Autodesk Inventor part; units mm, degrees
(part 2 of 2)
sketch "Sketch21" plane through (-13, -6, 11) normal (0, 0, 1) x (1, 0, 0)
  line L0 (3, 1.5332) -> (-3, 1.5332)
  arc A0 (3, 1.5332) -> (-3, 1.5332) centre (0, 0) ccw
  circle A1 centre (0, 0) radius 3.5 projected
  line L1 (2.0687, 0.6882) -> (2.0687, -0.0132) construction
  line L2 (2.0687, -0.0132) -> (1.4411, -0.0132) construction
  line L3 (1.4411, -0.0132) -> (1.4411, 0.6882) construction
  line L4 (1.4411, 0.6882) -> (2.0687, 0.6882) construction
  line L5 (11, 13.9476) -> (5, 13.9476)
  arc A2 (11, 13.9476) -> (5, 13.9476) centre (8, 12.4145) ccw
  line L6 (10.0687, 12.6882) -> (10.0687, 11.9868) construction
  line L7 (10.0687, 11.9868) -> (9.4411, 11.9868) construction
  line L8 (9.4411, 11.9868) -> (9.4411, 12.6882) construction
  line L9 (9.4411, 12.6882) -> (10.0687, 12.6882) construction
  line L10 (3, 1.5332) -> (-3, 1.5332)
  arc A3 (3, 1.5332) -> (-3, 1.5332) centre (0, 0) ccw
  line L11 (11, 13.9476) -> (5, 13.9476)
  arc A4 (11, 13.9476) -> (5, 13.9476) centre (8, 12.4145) ccw
  line L12 (1.0216, -0.0191) -> (1.0216, 0.6134)
  line L13 (1.0216, 0.6134) -> (1.1671, 0.6134)
  spline S0 degree 2 poles (1.1671, 0.6134) (1.2311, 0.5452) (1.3499, 0.4239) (1.4139, 0.3657) knots 0 0 0 1 2 2 2
  spline S1 degree 2 poles (1.4139, 0.3657) (1.5427, 0.2485) (1.6973, 0.1629) (1.7795, 0.1629) knots 0 0 0 1 2 2 2
  spline S2 degree 2 poles (1.7795, 0.1629) (1.8228, 0.1629) (1.8876, 0.1895) (1.9084, 0.2136) knots 0 0 0 1 2 2 2
  spline S3 degree 2 poles (1.9084, 0.2136) (1.9291, 0.2377) (1.9499, 0.3009) (1.9499, 0.3391) knots 0 0 0 1 2 2 2
  spline S4 degree 2 poles (1.9499, 0.3391) (1.9499, 0.3757) (1.9316, 0.4505) (1.9175, 0.4845) knots 0 0 0 1 2 2 2
  spline S5 degree 2 poles (1.9175, 0.4845) (1.9059, 0.5136) (1.8726, 0.5677) (1.861, 0.5843) knots 0 0 0 1 2 2 2
  line L14 (1.861, 0.5843) -> (1.861, 0.5918)
  line L15 (1.861, 0.5918) -> (2.0073, 0.5918)
  spline S6 degree 2 poles (2.0073, 0.5918) (2.028, 0.5494) (2.0687, 0.3973) (2.0687, 0.3291) knots 0 0 0 1 2 2 2
  spline S7 degree 2 poles (2.0687, 0.3291) (2.0687, 0.1854) (1.9167, 0.0233) (1.787, 0.0233) knots 0 0 0 1 2 2 2
  spline S8 degree 2 poles (1.787, 0.0233) (1.7264, 0.0233) (1.625, 0.0516) (1.5818, 0.0765) knots 0 0 0 1 2 2 2
  spline S9 degree 2 poles (1.5818, 0.0765) (1.5369, 0.1014) (1.4488, 0.1737) (1.4064, 0.2136) knots 0 0 0 1 2 2 2
  spline S10 degree 2 poles (1.4064, 0.2136) (1.3358, 0.2784) (1.1845, 0.4372) (1.1405, 0.4845) knots 0 0 0 1 2 2 2
  line L16 (1.1405, 0.4845) -> (1.1405, -0.0191)
  line L17 (1.1405, -0.0191) -> (1.0216, -0.0191)
  line L18 (1.0216, -0.7886) -> (1.0216, -0.1562)
  line L19 (1.0216, -0.1562) -> (1.1671, -0.1562)
  spline S11 degree 2 poles (1.1671, -0.1562) (1.2311, -0.2243) (1.3499, -0.3457) (1.4139, -0.4038) knots 0 0 0 1 2 2 2
  spline S12 degree 2 poles (1.4139, -0.4038) (1.5427, -0.521) (1.6973, -0.6066) (1.7795, -0.6066) knots 0 0 0 1 2 2 2
  spline S13 degree 2 poles (1.7795, -0.6066) (1.8228, -0.6066) (1.8876, -0.58) (1.9084, -0.5559) knots 0 0 0 1 2 2 2
  spline S14 degree 2 poles (1.9084, -0.5559) (1.9291, -0.5318) (1.9499, -0.4687) (1.9499, -0.4304) knots 0 0 0 1 2 2 2
  spline S15 degree 2 poles (1.9499, -0.4304) (1.9499, -0.3939) (1.9316, -0.3191) (1.9175, -0.285) knots 0 0 0 1 2 2 2
  spline S16 degree 2 poles (1.9175, -0.285) (1.9059, -0.2559) (1.8726, -0.2019) (1.861, -0.1853) knots 0 0 0 1 2 2 2
  line L20 (1.861, -0.1853) -> (1.861, -0.1778)
  line L21 (1.861, -0.1778) -> (2.0073, -0.1778)
  spline S17 degree 2 poles (2.0073, -0.1778) (2.028, -0.2202) (2.0687, -0.3723) (2.0687, -0.4404) knots 0 0 0 1 2 2 2
  spline S18 degree 2 poles (2.0687, -0.4404) (2.0687, -0.5842) (1.9167, -0.7462) (1.787, -0.7462) knots 0 0 0 1 2 2 2
  spline S19 degree 2 poles (1.787, -0.7462) (1.7264, -0.7462) (1.625, -0.718) (1.5818, -0.693) knots 0 0 0 1 2 2 2
  spline S20 degree 2 poles (1.5818, -0.693) (1.5369, -0.6681) (1.4488, -0.5958) (1.4064, -0.5559) knots 0 0 0 1 2 2 2
  spline S21 degree 2 poles (1.4064, -0.5559) (1.3358, -0.4911) (1.1845, -0.3324) (1.1405, -0.285) knots 0 0 0 1 2 2 2
  line L22 (1.1405, -0.285) -> (1.1405, -0.7886)
  line L23 (1.1405, -0.7886) -> (1.0216, -0.7886)
  spline S22 degree 2 poles (1.5344, -1.564) (1.2585, -1.564) (1, -1.4036) (1, -1.2365) knots 0 0 0 1 2 2 2
  spline S23 degree 2 poles (1, -1.2365) (1, -1.067) (1.2635, -0.9083) (1.5336, -0.9083) knots 0 0 0 1 2 2 2
  spline S24 degree 2 poles (1.5336, -0.9083) (1.8111, -0.9083) (2.0679, -1.0687) (2.0679, -1.2365) knots 0 0 0 1 2 2 2
  spline S25 degree 2 poles (2.0679, -1.2365) (2.0679, -1.4052) (1.802, -1.564) (1.5344, -1.564) knots 0 0 0 1 2 2 2
  spline S26 degree 2 poles (1.2219, -1.3878) (1.2726, -1.4077) (1.4288, -1.4243) (1.5344, -1.4243) knots 0 0 0 1 2 2 2
  spline S27 degree 2 poles (1.5344, -1.4243) (1.6399, -1.4243) (1.7953, -1.4077) (1.8477, -1.3869) knots 0 0 0 1 2 2 2
  spline S28 degree 2 poles (1.8477, -1.3869) (1.9, -1.3662) (1.9541, -1.2939) (1.9541, -1.2365) knots 0 0 0 1 2 2 2
  spline S29 degree 2 poles (1.9541, -1.2365) (1.9541, -1.1792) (1.9, -1.1052) (1.846, -1.0836) knots 0 0 0 1 2 2 2
  spline S30 degree 2 poles (1.846, -1.0836) (1.7937, -1.0628) (1.6341, -1.0479) (1.5336, -1.0479) knots 0 0 0 1 2 2 2
  spline S31 degree 2 poles (1.5336, -1.0479) (1.4255, -1.0479) (1.2809, -1.0612) (1.2244, -1.0828) knots 0 0 0 1 2 2 2
  spline S32 degree 2 poles (1.2244, -1.0828) (1.1712, -1.1027) (1.1139, -1.1767) (1.1139, -1.2365) knots 0 0 0 1 2 2 2
  spline S33 degree 2 poles (1.1139, -1.2365) (1.1139, -1.293) (1.1679, -1.367) (1.2219, -1.3878) knots 0 0 0 1 2 2 2
  spline S34 degree 2 poles (0.2615, 0.3366) (0.2615, 0.374) (0.2432, 0.448) (0.229, 0.4837) knots 0 0 0 1 2 2 2
  spline S35 degree 2 poles (0.229, 0.4837) (0.2149, 0.517) (0.185, 0.566) (0.1717, 0.5851) knots 0 0 0 1 2 2 2
  line L24 (0.1717, 0.5851) -> (0.1717, 0.5934)
  line L25 (0.1717, 0.5934) -> (0.3171, 0.5934)
  spline S36 degree 2 poles (0.3171, 0.5934) (0.3412, 0.5485) (0.3803, 0.3948) (0.3803, 0.3258) knots 0 0 0 1 2 2 2
  spline S37 degree 2 poles (0.3803, 0.3258) (0.3803, 0.256) (0.352, 0.1521) (0.3221, 0.1097) knots 0 0 0 1 2 2 2
  spline S38 degree 2 poles (0.3221, 0.1097) (0.2897, 0.0649) (0.1958, 0.0183) (0.1326, 0.0183) knots 0 0 0 1 2 2 2
  spline S39 degree 2 poles (0.1326, 0.0183) (0.0479, 0.0183) (-0.0801, 0.1297) (-0.0967, 0.2078) knots 0 0 0 1 2 2 2
  line L26 (-0.0967, 0.2078) -> (-0.1067, 0.2078)
  spline S40 degree 2 poles (-0.1067, 0.2078) (-0.1133, 0.1754) (-0.1433, 0.1014) (-0.1732, 0.0699) knots 0 0 0 1 2 2 2
  spline S41 degree 2 poles (-0.1732, 0.0699) (-0.2023, 0.0383) (-0.2953, -0.0016) (-0.3627, -0.0016) knots 0 0 0 1 2 2 2
  spline S42 degree 2 poles (-0.3627, -0.0016) (-0.4316, -0.0016) (-0.5488, 0.0458) (-0.5937, 0.089) knots 0 0 0 1 2 2 2
  spline S43 degree 2 poles (-0.5937, 0.089) (-0.6402, 0.1338) (-0.6884, 0.261) (-0.6884, 0.3416) knots 0 0 0 1 2 2 2
  spline S44 degree 2 poles (-0.6884, 0.3416) (-0.6884, 0.4189) (-0.651, 0.5701) (-0.6253, 0.6217) knots 0 0 0 1 2 2 2
  line L27 (-0.6253, 0.6217) -> (-0.4798, 0.6217)
  line L28 (-0.4798, 0.6217) -> (-0.4798, 0.6117)
  spline S45 degree 2 poles (-0.4798, 0.6117) (-0.5114, 0.5685) (-0.5696, 0.4222) (-0.5696, 0.3499) knots 0 0 0 1 2 2 2
  spline S46 degree 2 poles (-0.5696, 0.3499) (-0.5696, 0.3075) (-0.543, 0.2228) (-0.5122, 0.1945) knots 0 0 0 1 2 2 2
  spline S47 degree 2 poles (-0.5122, 0.1945) (-0.4815, 0.1671) (-0.4084, 0.138) (-0.3527, 0.138) knots 0 0 0 1 2 2 2
  spline S48 degree 2 poles (-0.3527, 0.138) (-0.297, 0.138) (-0.2247, 0.1704) (-0.2039, 0.1995) knots 0 0 0 1 2 2 2
  spline S49 degree 2 poles (-0.2039, 0.1995) (-0.1832, 0.2286) (-0.1674, 0.3075) (-0.1674, 0.3541) knots 0 0 0 1 2 2 2
  line L29 (-0.1674, 0.3541) -> (-0.1674, 0.4122)
  line L30 (-0.1674, 0.4122) -> (-0.0535, 0.4122)
  line L31 (-0.0535, 0.4122) -> (-0.0535, 0.3665)
  spline S50 degree 2 poles (-0.0535, 0.3665) (-0.0535, 0.2743) (0.0346, 0.1579) (0.1185, 0.1579) knots 0 0 0 1 2 2 2
  spline S51 degree 2 poles (0.1185, 0.1579) (0.1576, 0.1579) (0.2133, 0.1879) (0.2299, 0.212) knots 0 0 0 1 2 2 2
  spline S52 degree 2 poles (0.2299, 0.212) (0.2473, 0.2377) (0.2615, 0.3009) (0.2615, 0.3366) knots 0 0 0 1 2 2 2
  spline S53 degree 2 poles (-0.3411, -0.7778) (-0.415, -0.7778) (-0.5413, -0.7304) (-0.5879, -0.6872) knots 0 0 0 1 2 2 2
  spline S54 degree 2 poles (-0.5879, -0.6872) (-0.6344, -0.644) (-0.6884, -0.5152) (-0.6884, -0.4354) knots 0 0 0 1 2 2 2
  spline S55 degree 2 poles (-0.6884, -0.4354) (-0.6884, -0.3623) (-0.656, -0.2193) (-0.6303, -0.167) knots 0 0 0 1 2 2 2
  line L32 (-0.6303, -0.167) -> (-0.4848, -0.167)
  line L33 (-0.4848, -0.167) -> (-0.4848, -0.177)
  spline S56 degree 2 poles (-0.4848, -0.177) (-0.4965, -0.1927) (-0.5264, -0.2518) (-0.5397, -0.2875) knots 0 0 0 1 2 2 2
  spline S57 degree 2 poles (-0.5397, -0.2875) (-0.5538, -0.3282) (-0.5696, -0.3955) (-0.5696, -0.4379) knots 0 0 0 1 2 2 2
  spline S58 degree 2 poles (-0.5696, -0.4379) (-0.5696, -0.4795) (-0.5397, -0.5576) (-0.5073, -0.5858) knots 0 0 0 1 2 2 2
  spline S59 degree 2 poles (-0.5073, -0.5858) (-0.4765, -0.6116) (-0.3951, -0.6382) (-0.3402, -0.6382) knots 0 0 0 1 2 2 2
  spline S60 degree 2 poles (-0.3402, -0.6382) (-0.2854, -0.6382) (-0.2156, -0.6083) (-0.1923, -0.58) knots 0 0 0 1 2 2 2
  spline S61 degree 2 poles (-0.1923, -0.58) (-0.1665, -0.5509) (-0.1449, -0.4645) (-0.1449, -0.4121) knots 0 0 0 1 2 2 2
  spline S62 degree 2 poles (-0.1449, -0.4121) (-0.1449, -0.3556) (-0.1624, -0.2434) (-0.1699, -0.2094) knots 0 0 0 1 2 2 2
  line L34 (-0.1699, -0.2094) -> (0.3587, -0.2094)
  line L35 (0.3587, -0.2094) -> (0.3587, -0.772)
  line L36 (0.3587, -0.772) -> (0.2382, -0.772)
  line L37 (0.2382, -0.772) -> (0.2382, -0.3415)
  line L38 (0.2382, -0.3415) -> (-0.0352, -0.3415)
  spline S63 degree 2 poles (-0.0352, -0.3415) (-0.0319, -0.3664) (-0.0294, -0.4146) (-0.0294, -0.4346) knots 0 0 0 1 2 2 2
  spline S64 degree 2 poles (-0.0294, -0.4346) (-0.0294, -0.5135) (-0.0552, -0.6224) (-0.0934, -0.6723) knots 0 0 0 1 2 2 2
  spline S65 degree 2 poles (-0.0934, -0.6723) (-0.1316, -0.723) (-0.248, -0.7778) (-0.3411, -0.7778) knots 0 0 0 1 2 2 2
  line L39 (0.3587, -1.6986) -> (-0.6668, -1.3454)
  line L40 (-0.6668, -1.3454) -> (-0.6668, -1.1983)
  line L41 (-0.6668, -1.1983) -> (0.3587, -0.8451)
  line L42 (0.3587, -0.8451) -> (0.3587, -0.9914)
  line L43 (0.3587, -0.9914) -> (-0.4931, -1.2756)
  line L44 (-0.4931, -1.2756) -> (0.3587, -1.5598)
  line L45 (0.3587, -1.5598) -> (0.3587, -1.6986)
  spline S66 degree 2 poles (-2.3769, 0.2261) (-2.3769, 0.3167) (-2.3295, 0.4513) (-2.2821, 0.4987) knots 0 0 0 1 2 2 2
  spline S67 degree 2 poles (-2.2821, 0.4987) (-2.229, 0.5527) (-2.0794, 0.5967) (-1.9697, 0.5967) knots 0 0 0 1 2 2 2
  line L46 (-1.9697, 0.5967) -> (-1.3298, 0.5967)
  line L47 (-1.3298, 0.5967) -> (-1.3298, 0.4604)
  line L48 (-1.3298, 0.4604) -> (-1.9697, 0.4604)
  spline S68 degree 2 poles (-1.9697, 0.4604) (-2.0411, 0.4604) (-2.1375, 0.4422) (-2.1766, 0.4164) knots 0 0 0 1 2 2 2
  spline S69 degree 2 poles (-2.1766, 0.4164) (-2.2182, 0.389) (-2.2605, 0.2942) (-2.2605, 0.2261) knots 0 0 0 1 2 2 2
  spline S70 degree 2 poles (-2.2605, 0.2261) (-2.2605, 0.1621) (-2.2182, 0.0624) (-2.1766, 0.035) knots 0 0 0 1 2 2 2
  spline S71 degree 2 poles (-2.1766, 0.035) (-2.1375, 0.0092) (-2.042, -0.0091) (-1.973, -0.0091) knots 0 0 0 1 2 2 2
  line L49 (-1.973, -0.0091) -> (-1.3298, -0.0091)
  line L50 (-1.3298, -0.0091) -> (-1.3298, -0.1454)
  line L51 (-1.3298, -0.1454) -> (-1.9697, -0.1454)
  spline S72 degree 2 poles (-1.9697, -0.1454) (-2.0769, -0.1454) (-2.2298, -0.1022) (-2.2821, -0.0473) knots 0 0 0 1 2 2 2
  spline S73 degree 2 poles (-2.2821, -0.0473) (-2.3303, 0.0017) (-2.3769, 0.1314) (-2.3769, 0.2261) knots 0 0 0 1 2 2 2
  line L52 (-2.3553, -0.58) -> (-1.4511, -0.58)
  line L53 (-1.4511, -0.58) -> (-1.4511, -0.236)
  line L54 (-1.4511, -0.236) -> (-1.3298, -0.236)
  line L55 (-1.3298, -0.236) -> (-1.3298, -1.0604)
  line L56 (-1.3298, -1.0604) -> (-1.4511, -1.0604)
  line L57 (-1.4511, -1.0604) -> (-1.4511, -0.7163)
  line L58 (-1.4511, -0.7163) -> (-2.3553, -0.7163)
  line L59 (-2.3553, -0.7163) -> (-2.3553, -0.58)
  line L60 (9.0216, 11.9809) -> (9.0216, 12.6134)
  line L61 (9.0216, 12.6134) -> (9.1671, 12.6134)
  spline S74 degree 2 poles (9.1671, 12.6134) (9.2311, 12.5452) (9.3499, 12.4239) (9.4139, 12.3657) knots 0 0 0 1 2 2 2
  spline S75 degree 2 poles (9.4139, 12.3657) (9.5427, 12.2485) (9.6973, 12.1629) (9.7795, 12.1629) knots 0 0 0 1 2 2 2
  spline S76 degree 2 poles (9.7795, 12.1629) (9.8228, 12.1629) (9.8876, 12.1895) (9.9084, 12.2136) knots 0 0 0 1 2 2 2
  spline S77 degree 2 poles (9.9084, 12.2136) (9.9291, 12.2377) (9.9499, 12.3009) (9.9499, 12.3391) knots 0 0 0 1 2 2 2
  spline S78 degree 2 poles (9.9499, 12.3391) (9.9499, 12.3757) (9.9316, 12.4505) (9.9175, 12.4845) knots 0 0 0 1 2 2 2
  spline S79 degree 2 poles (9.9175, 12.4845) (9.9059, 12.5136) (9.8726, 12.5677) (9.861, 12.5843) knots 0 0 0 1 2 2 2
  line L62 (9.861, 12.5843) -> (9.861, 12.5918)
  line L63 (9.861, 12.5918) -> (10.0073, 12.5918)
  spline S80 degree 2 poles (10.0073, 12.5918) (10.028, 12.5494) (10.0687, 12.3973) (10.0687, 12.3291) knots 0 0 0 1 2 2 2
  spline S81 degree 2 poles (10.0687, 12.3291) (10.0687, 12.1854) (9.9167, 12.0233) (9.787, 12.0233) knots 0 0 0 1 2 2 2
  spline S82 degree 2 poles (9.787, 12.0233) (9.7264, 12.0233) (9.625, 12.0516) (9.5818, 12.0765) knots 0 0 0 1 2 2 2
  spline S83 degree 2 poles (9.5818, 12.0765) (9.5369, 12.1014) (9.4488, 12.1737) (9.4064, 12.2136) knots 0 0 0 1 2 2 2
  spline S84 degree 2 poles (9.4064, 12.2136) (9.3358, 12.2784) (9.1845, 12.4372) (9.1405, 12.4845) knots 0 0 0 1 2 2 2
  line L64 (9.1405, 12.4845) -> (9.1405, 11.9809)
  line L65 (9.1405, 11.9809) -> (9.0216, 11.9809)
  line L66 (9.0216, 11.2114) -> (9.0216, 11.8438)
  line L67 (9.0216, 11.8438) -> (9.1671, 11.8438)
  spline S85 degree 2 poles (9.1671, 11.8438) (9.2311, 11.7757) (9.3499, 11.6543) (9.4139, 11.5962) knots 0 0 0 1 2 2 2
  spline S86 degree 2 poles (9.4139, 11.5962) (9.5427, 11.479) (9.6973, 11.3934) (9.7795, 11.3934) knots 0 0 0 1 2 2 2
  spline S87 degree 2 poles (9.7795, 11.3934) (9.8228, 11.3934) (9.8876, 11.42) (9.9084, 11.4441) knots 0 0 0 1 2 2 2
  spline S88 degree 2 poles (9.9084, 11.4441) (9.9291, 11.4682) (9.9499, 11.5313) (9.9499, 11.5696) knots 0 0 0 1 2 2 2
  spline S89 degree 2 poles (9.9499, 11.5696) (9.9499, 11.6061) (9.9316, 11.6809) (9.9175, 11.715) knots 0 0 0 1 2 2 2
  spline S90 degree 2 poles (9.9175, 11.715) (9.9059, 11.7441) (9.8726, 11.7981) (9.861, 11.8147) knots 0 0 0 1 2 2 2
  line L68 (9.861, 11.8147) -> (9.861, 11.8222)
  line L69 (9.861, 11.8222) -> (10.0073, 11.8222)
  spline S91 degree 2 poles (10.0073, 11.8222) (10.028, 11.7798) (10.0687, 11.6277) (10.0687, 11.5596) knots 0 0 0 1 2 2 2
  spline S92 degree 2 poles (10.0687, 11.5596) (10.0687, 11.4158) (9.9167, 11.2538) (9.787, 11.2538) knots 0 0 0 1 2 2 2
  spline S93 degree 2 poles (9.787, 11.2538) (9.7264, 11.2538) (9.625, 11.282) (9.5818, 11.307) knots 0 0 0 1 2 2 2
  spline S94 degree 2 poles (9.5818, 11.307) (9.5369, 11.3319) (9.4488, 11.4042) (9.4064, 11.4441) knots 0 0 0 1 2 2 2
  spline S95 degree 2 poles (9.4064, 11.4441) (9.3358, 11.5089) (9.1845, 11.6676) (9.1405, 11.715) knots 0 0 0 1 2 2 2
  line L70 (9.1405, 11.715) -> (9.1405, 11.2114)
  line L71 (9.1405, 11.2114) -> (9.0216, 11.2114)
  spline S96 degree 2 poles (9.5344, 10.436) (9.2585, 10.436) (9, 10.5964) (9, 10.7635) knots 0 0 0 1 2 2 2
  spline S97 degree 2 poles (9, 10.7635) (9, 10.933) (9.2635, 11.0917) (9.5336, 11.0917) knots 0 0 0 1 2 2 2
  spline S98 degree 2 poles (9.5336, 11.0917) (9.8111, 11.0917) (10.0679, 10.9313) (10.0679, 10.7635) knots 0 0 0 1 2 2 2
  spline S99 degree 2 poles (10.0679, 10.7635) (10.0679, 10.5948) (9.802, 10.436) (9.5344, 10.436) knots 0 0 0 1 2 2 2
  spline S100 degree 2 poles (9.2219, 10.6122) (9.2726, 10.5923) (9.4288, 10.5757) (9.5344, 10.5757) knots 0 0 0 1 2 2 2
  spline S101 degree 2 poles (9.5344, 10.5757) (9.6399, 10.5757) (9.7953, 10.5923) (9.8477, 10.6131) knots 0 0 0 1 2 2 2
  spline S102 degree 2 poles (9.8477, 10.6131) (9.9, 10.6338) (9.9541, 10.7061) (9.9541, 10.7635) knots 0 0 0 1 2 2 2
  spline S103 degree 2 poles (9.9541, 10.7635) (9.9541, 10.8208) (9.9, 10.8948) (9.846, 10.9164) knots 0 0 0 1 2 2 2
  spline S104 degree 2 poles (9.846, 10.9164) (9.7937, 10.9372) (9.6341, 10.9521) (9.5336, 10.9521) knots 0 0 0 1 2 2 2
  spline S105 degree 2 poles (9.5336, 10.9521) (9.4255, 10.9521) (9.2809, 10.9388) (9.2244, 10.9172) knots 0 0 0 1 2 2 2
  spline S106 degree 2 poles (9.2244, 10.9172) (9.1712, 10.8973) (9.1139, 10.8233) (9.1139, 10.7635) knots 0 0 0 1 2 2 2
  spline S107 degree 2 poles (9.1139, 10.7635) (9.1139, 10.707) (9.1679, 10.633) (9.2219, 10.6122) knots 0 0 0 1 2 2 2
  spline S108 degree 2 poles (8.2615, 12.3366) (8.2615, 12.374) (8.2432, 12.448) (8.229, 12.4837) knots 0 0 0 1 2 2 2
  spline S109 degree 2 poles (8.229, 12.4837) (8.2149, 12.517) (8.185, 12.566) (8.1717, 12.5851) knots 0 0 0 1 2 2 2
  line L72 (8.1717, 12.5851) -> (8.1717, 12.5934)
  line L73 (8.1717, 12.5934) -> (8.3171, 12.5934)
  spline S110 degree 2 poles (8.3171, 12.5934) (8.3412, 12.5485) (8.3803, 12.3948) (8.3803, 12.3258) knots 0 0 0 1 2 2 2
  spline S111 degree 2 poles (8.3803, 12.3258) (8.3803, 12.256) (8.352, 12.1521) (8.3221, 12.1097) knots 0 0 0 1 2 2 2
  spline S112 degree 2 poles (8.3221, 12.1097) (8.2897, 12.0649) (8.1958, 12.0183) (8.1326, 12.0183) knots 0 0 0 1 2 2 2
  spline S113 degree 2 poles (8.1326, 12.0183) (8.0479, 12.0183) (7.9199, 12.1297) (7.9033, 12.2078) knots 0 0 0 1 2 2 2
  line L74 (7.9033, 12.2078) -> (7.8933, 12.2078)
  spline S114 degree 2 poles (7.8933, 12.2078) (7.8867, 12.1754) (7.8567, 12.1014) (7.8268, 12.0699) knots 0 0 0 1 2 2 2
  spline S115 degree 2 poles (7.8268, 12.0699) (7.7977, 12.0383) (7.7047, 11.9984) (7.6373, 11.9984) knots 0 0 0 1 2 2 2
  spline S116 degree 2 poles (7.6373, 11.9984) (7.5684, 11.9984) (7.4512, 12.0458) (7.4063, 12.089) knots 0 0 0 1 2 2 2
  spline S117 degree 2 poles (7.4063, 12.089) (7.3598, 12.1338) (7.3116, 12.261) (7.3116, 12.3416) knots 0 0 0 1 2 2 2
  spline S118 degree 2 poles (7.3116, 12.3416) (7.3116, 12.4189) (7.349, 12.5701) (7.3747, 12.6217) knots 0 0 0 1 2 2 2
  line L75 (7.3747, 12.6217) -> (7.5202, 12.6217)
  line L76 (7.5202, 12.6217) -> (7.5202, 12.6117)
  spline S119 degree 2 poles (7.5202, 12.6117) (7.4886, 12.5685) (7.4304, 12.4222) (7.4304, 12.3499) knots 0 0 0 1 2 2 2
  spline S120 degree 2 poles (7.4304, 12.3499) (7.4304, 12.3075) (7.457, 12.2228) (7.4878, 12.1945) knots 0 0 0 1 2 2 2
  spline S121 degree 2 poles (7.4878, 12.1945) (7.5185, 12.1671) (7.5916, 12.138) (7.6473, 12.138) knots 0 0 0 1 2 2 2
  spline S122 degree 2 poles (7.6473, 12.138) (7.703, 12.138) (7.7753, 12.1704) (7.7961, 12.1995) knots 0 0 0 1 2 2 2
  spline S123 degree 2 poles (7.7961, 12.1995) (7.8168, 12.2286) (7.8326, 12.3075) (7.8326, 12.3541) knots 0 0 0 1 2 2 2
  line L77 (7.8326, 12.3541) -> (7.8326, 12.4122)
  line L78 (7.8326, 12.4122) -> (7.9465, 12.4122)
  line L79 (7.9465, 12.4122) -> (7.9465, 12.3665)
  spline S124 degree 2 poles (7.9465, 12.3665) (7.9465, 12.2743) (8.0346, 12.1579) (8.1185, 12.1579) knots 0 0 0 1 2 2 2
  spline S125 degree 2 poles (8.1185, 12.1579) (8.1576, 12.1579) (8.2133, 12.1879) (8.2299, 12.212) knots 0 0 0 1 2 2 2
  spline S126 degree 2 poles (8.2299, 12.212) (8.2473, 12.2377) (8.2615, 12.3009) (8.2615, 12.3366) knots 0 0 0 1 2 2 2
  spline S127 degree 2 poles (7.6589, 11.2222) (7.585, 11.2222) (7.4587, 11.2696) (7.4121, 11.3128) knots 0 0 0 1 2 2 2
  spline S128 degree 2 poles (7.4121, 11.3128) (7.3656, 11.356) (7.3116, 11.4848) (7.3116, 11.5646) knots 0 0 0 1 2 2 2
  spline S129 degree 2 poles (7.3116, 11.5646) (7.3116, 11.6377) (7.344, 11.7807) (7.3697, 11.833) knots 0 0 0 1 2 2 2
  line L80 (7.3697, 11.833) -> (7.5152, 11.833)
  line L81 (7.5152, 11.833) -> (7.5152, 11.823)
  spline S130 degree 2 poles (7.5152, 11.823) (7.5035, 11.8073) (7.4736, 11.7482) (7.4603, 11.7125) knots 0 0 0 1 2 2 2
  spline S131 degree 2 poles (7.4603, 11.7125) (7.4462, 11.6718) (7.4304, 11.6045) (7.4304, 11.5621) knots 0 0 0 1 2 2 2
  spline S132 degree 2 poles (7.4304, 11.5621) (7.4304, 11.5205) (7.4603, 11.4424) (7.4927, 11.4142) knots 0 0 0 1 2 2 2
  spline S133 degree 2 poles (7.4927, 11.4142) (7.5235, 11.3884) (7.6049, 11.3618) (7.6598, 11.3618) knots 0 0 0 1 2 2 2
  spline S134 degree 2 poles (7.6598, 11.3618) (7.7146, 11.3618) (7.7844, 11.3917) (7.8077, 11.42) knots 0 0 0 1 2 2 2
  spline S135 degree 2 poles (7.8077, 11.42) (7.8335, 11.4491) (7.8551, 11.5355) (7.8551, 11.5879) knots 0 0 0 1 2 2 2
  spline S136 degree 2 poles (7.8551, 11.5879) (7.8551, 11.6444) (7.8376, 11.7566) (7.8301, 11.7906) knots 0 0 0 1 2 2 2
  line L82 (7.8301, 11.7906) -> (8.3587, 11.7906)
  line L83 (8.3587, 11.7906) -> (8.3587, 11.228)
  line L84 (8.3587, 11.228) -> (8.2382, 11.228)
  line L85 (8.2382, 11.228) -> (8.2382, 11.6585)
  line L86 (8.2382, 11.6585) -> (7.9648, 11.6585)
  spline S137 degree 2 poles (7.9648, 11.6585) (7.9681, 11.6336) (7.9706, 11.5854) (7.9706, 11.5654) knots 0 0 0 1 2 2 2
  spline S138 degree 2 poles (7.9706, 11.5654) (7.9706, 11.4865) (7.9448, 11.3776) (7.9066, 11.3277) knots 0 0 0 1 2 2 2
  spline S139 degree 2 poles (7.9066, 11.3277) (7.8684, 11.277) (7.752, 11.2222) (7.6589, 11.2222) knots 0 0 0 1 2 2 2
  line L87 (8.3587, 10.3014) -> (7.3332, 10.6546)
  line L88 (7.3332, 10.6546) -> (7.3332, 10.8017)
  line L89 (7.3332, 10.8017) -> (8.3587, 11.1549)
  line L90 (8.3587, 11.1549) -> (8.3587, 11.0086)
  line L91 (8.3587, 11.0086) -> (7.5069, 10.7244)
  line L92 (7.5069, 10.7244) -> (8.3587, 10.4402)
  line L93 (8.3587, 10.4402) -> (8.3587, 10.3014)
  spline S140 degree 2 poles (5.6231, 12.2261) (5.6231, 12.3167) (5.6705, 12.4513) (5.7179, 12.4987) knots 0 0 0 1 2 2 2
  spline S141 degree 2 poles (5.7179, 12.4987) (5.771, 12.5527) (5.9206, 12.5967) (6.0303, 12.5967) knots 0 0 0 1 2 2 2
  line L94 (6.0303, 12.5967) -> (6.6702, 12.5967)
  line L95 (6.6702, 12.5967) -> (6.6702, 12.4604)
  line L96 (6.6702, 12.4604) -> (6.0303, 12.4604)
  spline S142 degree 2 poles (6.0303, 12.4604) (5.9589, 12.4604) (5.8625, 12.4422) (5.8234, 12.4164) knots 0 0 0 1 2 2 2
  spline S143 degree 2 poles (5.8234, 12.4164) (5.7818, 12.389) (5.7395, 12.2942) (5.7395, 12.2261) knots 0 0 0 1 2 2 2
  spline S144 degree 2 poles (5.7395, 12.2261) (5.7395, 12.1621) (5.7818, 12.0624) (5.8234, 12.035) knots 0 0 0 1 2 2 2
  spline S145 degree 2 poles (5.8234, 12.035) (5.8625, 12.0092) (5.958, 11.9909) (6.027, 11.9909) knots 0 0 0 1 2 2 2
  line L97 (6.027, 11.9909) -> (6.6702, 11.9909)
  line L98 (6.6702, 11.9909) -> (6.6702, 11.8546)
  line L99 (6.6702, 11.8546) -> (6.0303, 11.8546)
  spline S146 degree 2 poles (6.0303, 11.8546) (5.9231, 11.8546) (5.7702, 11.8978) (5.7179, 11.9527) knots 0 0 0 1 2 2 2
  spline S147 degree 2 poles (5.7179, 11.9527) (5.6697, 12.0017) (5.6231, 12.1314) (5.6231, 12.2261) knots 0 0 0 1 2 2 2
  line L100 (5.6447, 11.42) -> (6.5489, 11.42)
  line L101 (6.5489, 11.42) -> (6.5489, 11.764)
  line L102 (6.5489, 11.764) -> (6.6702, 11.764)
  line L103 (6.6702, 11.764) -> (6.6702, 10.9396)
  line L104 (6.6702, 10.9396) -> (6.5489, 10.9396)
  line L105 (6.5489, 10.9396) -> (6.5489, 11.2837)
  line L106 (6.5489, 11.2837) -> (5.6447, 11.2837)
  line L107 (5.6447, 11.2837) -> (5.6447, 11.42)
  point P0 (13, 6)
  constraints: 8 end point, 8 point on circle, 4 centre point, 2 collinear, 2 concentric, 2 horizontal, 4 other
extrude "Extrusion24" add sketch "Sketch21" along normal blind 0.0001 contours L0 A0 | L5 A2 | L12 L13 S0 S1 S2 S3 S4 S5 L14 L15 S6 S7 S8 S9 S10 L16 L17 | L18 L19 S11 S12 S13 S14 S15 S16 L20 L21 S17 S18 S19 S20 S21 L22 L23 | S22 S23 S24 S25 | S34 S35 L24 L25 S36 S37 S38 S39 L26 S40 S41 S42 S43 S44 L27 L28 S45 S46 S47 S48 S49 L29 L30 L31 S50 S51 S52 | S53 S54 S55 L32 L33 S56 S57 S58 S59 S60 S61 S62 L34 L35 L36 L37 L38 S63 S64 S65 | L39 L40 L41 L42 L43 L44 L45 | S66 S67 L46 L47 L48 S68 S69 S70 S71 L49 L50 L51 S72 S73 | L52 L53 L54 L55 L56 L57 L58 L59 | L60 L61 S74 S75 S76 S77 S78 S79 L62 L63 S80 S81 S82 S83 S84 L64 L65 | L66 L67 S85 S86 S87 S88 S89 S90 L68 L69 S91 S92 S93 S94 S95 L70 L71 | S96 S97 S98 S99 | S108 S109 L72 L73 S110 S111 S112 S113 L74 S114 S115 S116 S117 S118 L75 L76 S119 S120 S121 S122 S123 L77 L78 L79 S124 S125 S126 | S127 S128 S129 L80 L81 S130 S131 S132 S133 S134 S135 S136 L82 L83 L84 L85 L86 S137 S138 S139 | L87 L88 L89 L90 L91 L92 L93 | S140 S141 L94 L95 L96 S142 S143 S144 S145 L97 L98 L99 S146 S147 | L100 L101 L102 L103 L104 L105 L106 L107
extrude "Extrusion25" add sketch "Sketch6" along normal blind 2 contours L173 L172 L171 L170
body "Solid1"
